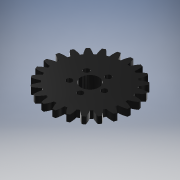
# Autodesk Inventor part: Spur Gear1
Saved by Autodesk Inventor 2017 SP1 (Build 210196100, 196)
## iProperties
Created: 2019-10-27
Part Number: Spur Gear1
Material: ABS Plastic
Document SubType Name: Modeling
Designer: Zach
Categories: <?xml version="1.0" encoding="UTF-16"?> <MemberInstance><Categories><FamilyTemplate><FamilyTemplateParameter ValueType="xs:double" Id="1" ObjectReferenceKey="da_z" ObjectType="kUserParameterObject"/><FamilyTemplateParameter ValueType="xs:double" Id="2" ObjectReferenceKey="da_b" ObjectType="kUserParameterObject"/><FamilyTemplateParameter ValueType="xs:double" Id="3" ObjectReferenceKey="da_beta" ObjectType="kUserParameterObject"/><FamilyTemplateParameter ValueType="xs:double" Id="4" ObjectReferenceKey="da_da" ObjectType="kUserParameterObject"/><FamilyTemplateParameter ValueType="xs:double" Id="5" ObjectReferenceKey="da_aw" ObjectType="kUserParameterObject"/><FamilyTemplateParameter ValueType="xs:string" Id="6" ObjectReferenceKey="EAIAABAAAACIAQAAAAAAAIAAAAAAAAAA" ObjectType="83910656" SubObjectId="SurfaceGeometry"/></FamilyTemplate><ParamToTemplateMap><ParamToTemplate CategoryParameter="//CategoryParameter[@InternalName='046C89C9-8512-4d59-83FE-43B91F4F132A']" TemplateParameter="1"/><ParamToTemplate CategoryParameter="//CategoryParameter[@InternalName='2552DF32-E462-4b46-AEBF-C6C7768E72AC']" TemplateParameter="2"/><ParamToTemplate CategoryParameter="//CategoryParameter[@InternalName='C9EE641D-15FC-4fae-A226-E94C4372FDD7']" TemplateParameter="3"/><ParamToTemplate><ParamToTemplate CategoryParameter="//CategoryParameter[@InternalName='00B6519A-459B-49c7-AD84-2E56D39A5744']" ConstantValue="0.000000"/></ParamToTemplate><ParamToTemplate><ParamToTemplate CategoryParameter="//CategoryParameter[@InternalName='04B31F0E-C7A6-4894-AA32-9629BEFACF47']" ConstantValue="1.000000"/></ParamToTemplate><ParamToTemplate><ParamToTemplate CategoryParameter="//CategoryParameter[@InternalName='43CBEC2E-7847-49e7-A936-2F7889FCB2D9']" ConstantValue="0.250000"/></ParamToTemplate><ParamToTemplate><ParamToTemplate CategoryParameter="//CategoryParameter[@InternalName='B1EFC894-105D-4ebd-86BF-FA20ED196853']" ConstantValue="0.350000"/></ParamToTemplate><ParamToTemplate><ParamToTemplate CategoryParameter="//CategoryParameter[@InternalName='51175063-3D10-4879-93E8-6246FE8B403D']" ConstantValue="2060000000.000000"/></ParamToTemplate><ParamToTemplate><ParamToTemplate CategoryParameter="//CategoryParameter[@InternalName='A3A52E27-4454-46a9-B0BD-C932399B70AF']" ConstantValue="0.300000"/></ParamToTemplate><ParamToTemplate><ParamToTemplate CategoryParameter="//CategoryParameter[@InternalName='91B76062-C214-41d9-B1B9-14D2AB99603D']" ConstantValue="0.150000"/></ParamToTemplate><ParamToTemplate><ParamToTemplate CategoryParameter="//CategoryParameter[@InternalName='374E806E-8B8A-4dda-A9AA-1039D6500AD2']" ConstantValue="6.666667"/></ParamToTemplate><ParamToTemplate><ParamToTemplate CategoryParameter="//CategoryParameter[@InternalName='2D373A89-B862-43d6-8D0B-0CBF12AB9F6C']" ConstantValue="0.392699"/></ParamToTemplate><ParamToTemplate CategoryParameter="//CategoryParameter[@InternalName='37777632-D6A2-4fac-9D53-DB8ACD95C989']" TemplateParameter="4"/><ParamToTemplate CategoryParameter="//CategoryParameter[@InternalName='FD1017F1-B727-4f7e-9707-0F86F1FF9423']" TemplateParameter="5"/><ParamToTemplate><ParamToTemplate CategoryParameter="//CategoryParameter[@InternalName='9E1B4470-B2D3-4ff1-B813-535BB4CDF51A']" ConstantValue="3520000.000000"/></ParamToTemplate><ParamToTemplate><ParamToTemplate CategoryParameter="//CategoryParameter[@InternalName='F8452263-BFF6-458c-9FB1-07C4B99E95CD']" ConstantValue="11400000.000000"/></ParamToTemplate><ParamToTemplate><ParamToTemplate CategoryParameter="//CategoryParameter[@InternalName='3E3BB259-FD49-497f-8171-6EBC954A3479']" ConstantValue="2.000000"/></ParamToTemplate><ParamToTemplate CategoryParameter="//CategoryParameter[@InternalName='27C3BAF2-7550-4e4b-AE2C-0DB134B7D9B7']" TemplateParameter="6"/></ParamToTemplateMap><Category DisplayName="Gear" InternalName="DC85795E-93AB-48d5-8EEE-5A27447B64BD" Mnemonic="Gear"><CategoryParameter DisplayName="z" InternalName="046C89C9-8512-4d59-83FE-43B91F4F132A" Mnemonic="z"/><CategoryParameter DisplayName="b" InternalName="2552DF32-E462-4b46-AEBF-C6C7768E72AC" Mnemonic="b"/><CategoryParameter DisplayName="||b|" InternalName="C9EE641D-15FC-4fae-A226-E94C4372FDD7" Mnemonic="beta"/><CategoryParameter DisplayName="x" InternalName="00B6519A-459B-49c7-AD84-2E56D39A5744" Mnemonic="x"/><CategoryParameter DisplayName="a*" InternalName="04B31F0E-C7A6-4894-AA32-9629BEFACF47" Mnemonic="a"/><CategoryParameter DisplayName="c*" InternalName="43CBEC2E-7847-49e7-A936-2F7889FCB2D9" Mnemonic="c"/><CategoryParameter DisplayName="r|.f|*" InternalName="B1EFC894-105D-4ebd-86BF-FA20ED196853" Mnemonic="rf"/><CategoryParameter DisplayName="E" InternalName="51175063-3D10-4879-93E8-6246FE8B403D" Mnemonic="E"/><CategoryParameter DisplayName="||m|" InternalName="A3A52E27-4454-46a9-B0BD-C932399B70AF" Mnemonic="mi"/><Category DisplayName="SpurGear" InternalName="26C5A22E-A91E-4dfd-A3B3-23CCAFAE1764" Mnemonic="SpurGear"><CategoryParameter DisplayName="m" InternalName="91B76062-C214-41d9-B1B9-14D2AB99603D" Mnemonic="m"/><CategoryParameter DisplayName="P" InternalName="374E806E-8B8A-4dda-A9AA-1039D6500AD2" Mnemonic="PP"/><CategoryParameter DisplayName="||a|" InternalName="2D373A89-B862-43d6-8D0B-0CBF12AB9F6C" Mnemonic="alpha"/><CategoryParameter DisplayName="d|.a|" InternalName="37777632-D6A2-4fac-9D53-DB8ACD95C989" Mnemonic="da"/><CategoryParameter DisplayName="a|.w|" InternalName="FD1017F1-B727-4f7e-9707-0F86F1FF9423" Mnemonic="aw"/><CategoryParameter DisplayName="||s||.Flim|" InternalName="9E1B4470-B2D3-4ff1-B813-535BB4CDF51A" Mnemonic="sFlim"/><CategoryParameter DisplayName="||s||.Hlim|" InternalName="F8452263-BFF6-458c-9FB1-07C4B99E95CD" Mnemonic="sHlim"/><CategoryParameter DisplayName="type" InternalName="3E3BB259-FD49-497f-8171-6EBC954A3479" Mnemonic="type"/><CategoryParameter DisplayName="PitchDiameter" InternalName="27C3BAF2-7550-4e4b-AE2C-0DB134B7D9B7" Mnemonic="IDS_PITCHDIAM"/></Category></Category></Categories></MemberInstance>
Density: 1.06 g/cm^3
Appearance: Smooth - Black
CustomPartVersion: 1
Author: Zach
Autodesk Inventor part; units mm, degrees
ref_plane "YZ Plane" through (0, 0, 0) normal (1, 0, 0) x (0, 1, 0)
ref_plane "XZ Plane" through (0, 0, 0) normal (0, 1, 0) x (-1, 0, 0)
ref_plane "XY Plane" through (0, 0, 0) normal (0, 0, 1) x (1, 0, 0)
sketch "Sketch1" plane through (0, 0, 0) normal (0, 0, 1) x (1, 0, 0)
  circle A0 centre (0, 0) radius 18.7297
  dimension "d0" = 37.4594
  constraints: 1 centre point
  measures "d0" diameter of A0
extrude "Extrusion1" add sketch "Sketch1" along normal blind 3
ref_plane "Work Plane2" through (0, 0, 1.5) normal (0, 0, 1) x (1, 0, 0)
sketch "Sketch2" plane through (0, 0, 0) normal (0, 0, -1) x (-1, 0, 0)
  circle A0 centre (0, 0) radius 18.7297 projected
  circle A1 centre (0, 0) radius 17.5
  dimension "d3" = 35
  constraints: 1 centre point, 1 coincident
  measures "d3" diameter of A1
surface extrude "Pitch Diameter" sketch "Sketch2" against normal through all shown no curves A1
ref_plane "Work Plane8" through (0, 0, 0) normal (0.9906859, 0.1361666, 0) x (0, 0, 1)
ref_plane "Work Plane9" through (0, 0, 0) normal (1, 0, 0) x (0, 1, 0)
spur gear teeth "Spur Gear" teeth 23 pitch diameter 34.5 tip diameter 37.4595 root diameter 30.75 face width 3 start plane through (0, 0, 0) normal (0, 0, -1) x (-1, 0, 0)
sketch "Sketch3" plane through (0, 0, 3) normal (0, 0, 1) x (1, 0, 0)
  circle A0 centre (0, 0) radius 4
  circle A1 centre (6.5, 0) radius 1.25
  circle A2 centre (2.0086, 6.1819) radius 1.25
  circle A3 centre (-5.2586, 3.8206) radius 1.25
  circle A4 centre (-5.2586, -3.8206) radius 1.25
  circle A5 centre (2.0086, -6.1819) radius 1.25
  dimension "d49" = 8
  dimension "d50" = 2.5
  dimension "d51" = 6.5
  dimension "d54" = 360
  constraints: 6 centre point, 1 coincident, 1 horizontal alignment, 11 other
  measures "d49" diameter of A0
  measures "d50" diameter of A1
  measures "d51" distance of A1.centre point (0, 0)
extrude "Extrusion2" cut sketch "Sketch3" against normal through all
sketch "Sketch4" plane through (0, 0, 0) normal (0, 0, -1) x (-1, 0, 0)
  circle A0 centre (0, 0) radius 11.5
  circle A1 centre (-2.0086, -6.1819) radius 1.25 projected
  circle A2 centre (5.2586, 3.8206) radius 1.25 projected
  circle A3 centre (-6.5, 0) radius 1.25 projected
  circle A4 centre (-2.0086, 6.1819) radius 1.25 projected
  circle A5 centre (5.2586, -3.8206) radius 1.25 projected
  circle A6 centre (0, 0) radius 4 projected
  arc A7 (5.6404, 14.303) -> (5.666, 17.8521) centre (-7.4576, 16.1723) ccw projected
  arc A8 (5.666, 17.8521) -> (4.4345, 18.1972) centre (0, 0) ccw projected
  arc A9 (4.4345, 18.1972) -> (2.6124, 15.1514) centre (14.7748, 9.943) ccw projected
  arc A10 (2.6124, 15.1514) -> (1.5723, 15.2944) centre (0, 0) ccw projected
  arc A11 (1.5723, 15.2944) -> (0.6395, 18.7188) centre (-11.5443, 13.5605) ccw projected
  arc A12 (0.6395, 18.7188) -> (-0.6395, 18.7188) centre (0, 0) ccw projected
  arc A13 (-0.6395, 18.7188) -> (-1.5723, 15.2944) centre (11.5443, 13.5605) ccw projected
  arc A14 (-1.5723, 15.2944) -> (-2.6124, 15.1514) centre (0, 0) ccw projected
  arc A15 (-2.6124, 15.1514) -> (-4.4345, 18.1972) centre (-14.7748, 9.943) ccw projected
  arc A16 (-4.4345, 18.1972) -> (-5.666, 17.8521) centre (0, 0) ccw projected
  arc A17 (-5.666, 17.8521) -> (-5.6404, 14.303) centre (7.4576, 16.1723) ccw projected
  arc A18 (-5.6404, 14.303) -> (-6.6033, 13.8848) centre (0, 0) ccw projected
  arc A19 (-6.6033, 13.8848) -> (-9.1796, 16.326) centre (-16.9095, 5.5881) ccw projected
  arc A20 (-9.1796, 16.326) -> (-10.2724, 15.6615) centre (0, 0) ccw projected
  arc A21 (-10.2724, 15.6615) -> (-9.2901, 12.2509) centre (2.8178, 17.5846) ccw projected
  arc A22 (-9.2901, 12.2509) -> (-10.1045, 11.5883) centre (0, 0) ccw projected
  arc A23 (-10.1045, 11.5883) -> (-13.2439, 13.2439) centre (-17.7901, 0.8188) ccw projected
  arc A24 (-13.2439, 13.2439) -> (-14.1168, 12.3092) centre (0, 0) ccw projected
  arc A25 (-14.1168, 12.3092) -> (-12.2509, 9.2901) centre (-2.0309, 17.6928) ccw projected
  arc A26 (-12.2509, 9.2901) -> (-12.8563, 8.4324) centre (0, 0) ccw projected
  arc A27 (-12.8563, 8.4324) -> (-16.326, 9.1796) centre (-17.3513, -4.0113) ccw projected
  arc A28 (-16.326, 9.1796) -> (-16.9143, 8.0441) centre (0, 0) ccw projected
  arc A29 (-16.9143, 8.0441) -> (-14.303, 5.6404) centre (-6.7291, 16.4887) ccw projected
  arc A30 (-14.303, 5.6404) -> (-14.6546, 4.6512) centre (0, 0) ccw projected
  arc A31 (-14.6546, 4.6512) -> (-18.1972, 4.4345) centre (-15.6256, -8.5439) ccw projected
  arc A32 (-18.1972, 4.4345) -> (-18.4574, 3.1824) centre (0, 0) ccw projected
  arc A33 (-18.4574, 3.1824) -> (-15.2944, 1.5723) centre (-10.9281, 14.0618) ccw projected
  arc A34 (-15.2944, 1.5723) -> (-15.366, 0.5249) centre (0, 0) ccw projected
  arc A35 (-15.366, 0.5249) -> (-18.7188, -0.6395) centre (-12.7411, -12.4428) ccw projected
  arc A36 (-18.7188, -0.6395) -> (-18.6315, -1.9154) centre (0, 0) ccw projected
  arc A37 (-18.6315, -1.9154) -> (-15.1514, -2.6124) centre (-14.3167, 10.592) ccw projected
  arc A38 (-15.1514, -2.6124) -> (-14.9378, -3.6403) centre (0, 0) ccw projected
  arc A39 (-14.9378, -3.6403) -> (-17.8521, -5.666) centre (-8.9116, -15.4189) ccw projected
  arc A40 (-17.8521, -5.666) -> (-17.4239, -6.8711) centre (0, 0) ccw projected
  arc A41 (-17.4239, -6.8711) -> (-13.8848, -6.6033) centre (-16.6435, 6.3366) ccw projected
  arc A42 (-13.8848, -6.6033) -> (-13.4018, -7.5354) centre (0, 0) ccw projected
  arc A43 (-13.4018, -7.5354) -> (-15.6615, -10.2724) centre (-4.4212, -17.2514) ccw projected
  arc A44 (-15.6615, -10.2724) -> (-14.9239, -11.3172) centre (0, 0) ccw projected
  arc A45 (-14.9239, -11.3172) -> (-11.5883, -10.1045) centre (-17.7359, 1.6112) ccw projected
  arc A46 (-11.5883, -10.1045) -> (-10.8718, -10.8718) centre (0, 0) ccw projected
  arc A47 (-10.8718, -10.8718) -> (-12.3092, -14.1168) centre (0.3972, -17.8045) ccw projected
  arc A48 (-12.3092, -14.1168) -> (-11.3172, -14.9239) centre (0, 0) ccw projected
  arc A49 (-11.3172, -14.9239) -> (-8.4324, -12.8563) centre (-17.5129, -3.2336) ccw projected
  arc A50 (-8.4324, -12.8563) -> (-7.5354, -13.4018) centre (0, 0) ccw projected
  arc A51 (-7.5354, -13.4018) -> (-8.0441, -16.9143) centre (5.186, -17.0371) ccw projected
  arc A52 (-8.0441, -16.9143) -> (-6.8711, -17.4239) centre (0, 0) ccw projected
  arc A53 (-6.8711, -17.4239) -> (-4.6512, -14.6546) centre (-15.9911, -7.8386) ccw projected
  arc A54 (-4.6512, -14.6546) -> (-3.6403, -14.9378) centre (0, 0) ccw projected
  arc A55 (-3.6403, -14.9378) -> (-3.1824, -18.4574) centre (9.5903, -15.0062) ccw projected
  arc A56 (-3.1824, -18.4574) -> (-1.9154, -18.6315) centre (0, 0) ccw projected
  arc A57 (-1.9154, -18.6315) -> (-0.5249, -15.366) centre (-13.2833, -11.8623) ccw projected
  arc A58 (-0.5249, -15.366) -> (0.5249, -15.366) centre (0, 0) ccw projected
  arc A59 (0.5249, -15.366) -> (1.9154, -18.6315) centre (13.2833, -11.8623) ccw projected
  arc A60 (1.9154, -18.6315) -> (3.1824, -18.4574) centre (0, 0) ccw projected
  arc A61 (3.1824, -18.4574) -> (3.6403, -14.9378) centre (-9.5903, -15.0062) ccw projected
  arc A62 (3.6403, -14.9378) -> (4.6512, -14.6546) centre (0, 0) ccw projected
  arc A63 (4.6512, -14.6546) -> (6.8711, -17.4239) centre (15.9911, -7.8386) ccw projected
  arc A64 (6.8711, -17.4239) -> (8.0441, -16.9143) centre (0, 0) ccw projected
  arc A65 (8.0441, -16.9143) -> (7.5354, -13.4018) centre (-5.186, -17.0371) ccw projected
  arc A66 (7.5354, -13.4018) -> (8.4324, -12.8563) centre (0, 0) ccw projected
  arc A67 (8.4324, -12.8563) -> (11.3172, -14.9239) centre (17.5129, -3.2336) ccw projected
  arc A68 (11.3172, -14.9239) -> (12.3092, -14.1168) centre (0, 0) ccw projected
  arc A69 (12.3092, -14.1168) -> (10.8718, -10.8718) centre (-0.3972, -17.8045) ccw projected
  arc A70 (10.8718, -10.8718) -> (11.5883, -10.1045) centre (0, 0) ccw projected
  arc A71 (11.5883, -10.1045) -> (14.9239, -11.3172) centre (17.7359, 1.6112) ccw projected
  arc A72 (14.9239, -11.3172) -> (15.6615, -10.2724) centre (0, 0) ccw projected
  arc A73 (15.6615, -10.2724) -> (13.4018, -7.5354) centre (4.4212, -17.2514) ccw projected
  arc A74 (13.4018, -7.5354) -> (13.8848, -6.6033) centre (0, 0) ccw projected
  arc A75 (13.8848, -6.6033) -> (17.4239, -6.8711) centre (16.6435, 6.3366) ccw projected
  arc A76 (17.4239, -6.8711) -> (17.8521, -5.666) centre (0, 0) ccw projected
  arc A77 (17.8521, -5.666) -> (14.9378, -3.6403) centre (8.9116, -15.4189) ccw projected
  arc A78 (14.9378, -3.6403) -> (15.1514, -2.6124) centre (0, 0) ccw projected
  arc A79 (15.1514, -2.6124) -> (18.6315, -1.9154) centre (14.3167, 10.592) ccw projected
  arc A80 (18.6315, -1.9154) -> (18.7188, -0.6395) centre (0, 0) ccw projected
  arc A81 (18.7188, -0.6395) -> (15.366, 0.5249) centre (12.7411, -12.4428) ccw projected
  arc A82 (15.366, 0.5249) -> (15.2944, 1.5723) centre (0, 0) ccw projected
  arc A83 (15.2944, 1.5723) -> (18.4574, 3.1824) centre (10.9281, 14.0618) ccw projected
  arc A84 (18.4574, 3.1824) -> (18.1972, 4.4345) centre (0, 0) ccw projected
  arc A85 (18.1972, 4.4345) -> (14.6546, 4.6512) centre (15.6256, -8.5439) ccw projected
  arc A86 (14.6546, 4.6512) -> (14.303, 5.6404) centre (0, 0) ccw projected
  arc A87 (14.303, 5.6404) -> (16.9143, 8.0441) centre (6.7291, 16.4887) ccw projected
  arc A88 (16.9143, 8.0441) -> (16.326, 9.1796) centre (0, 0) ccw projected
  arc A89 (16.326, 9.1796) -> (12.8563, 8.4324) centre (17.3513, -4.0113) ccw projected
  arc A90 (12.8563, 8.4324) -> (12.2509, 9.2901) centre (0, 0) ccw projected
  arc A91 (12.2509, 9.2901) -> (14.1168, 12.3092) centre (2.0309, 17.6928) ccw projected
  arc A92 (14.1168, 12.3092) -> (13.2439, 13.2439) centre (0, 0) ccw projected
  arc A93 (13.2439, 13.2439) -> (10.1045, 11.5883) centre (17.7901, 0.8188) ccw projected
  arc A94 (10.1045, 11.5883) -> (9.2901, 12.2509) centre (0, 0) ccw projected
  arc A95 (9.2901, 12.2509) -> (10.2724, 15.6615) centre (-2.8178, 17.5846) ccw projected
  arc A96 (10.2724, 15.6615) -> (9.1796, 16.326) centre (0, 0) ccw projected
  arc A97 (9.1796, 16.326) -> (6.6033, 13.8848) centre (16.9095, 5.5881) ccw projected
  arc A98 (6.6033, 13.8848) -> (5.6404, 14.303) centre (0, 0) ccw projected
  dimension "d58" = 23
  constraints: 1 centre point, 1 coincident
  measures "d58" diameter of A0
extrude "Extrusion3" add sketch "Sketch4" along normal blind 3 contours A0
equation "\"d0\" = da_da"
equation "\"d1\" = da_b"
equation "\"d3\" = da_dw"
equation "\"d16\" = da_aw"
equation "\"d43\" = da_aw"
equation "\"d46\" = da_aw"
equation "\"da_da\" = 37.459454"
equation "\"da_b\" = 3"
equation "\"da_dw\" = 35"
equation "\"da_aw\" = 35"
body "Solid1"
body "Srf1"
